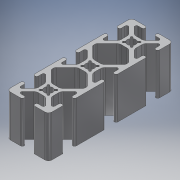
# Autodesk Inventor part: 1030-S
Saved by Autodesk Inventor 2017 SP1 (Build 210196100, 196)
## iProperties
Created: 2016-09-13
Part Number: 1030-S
Material: 6105-T5
Description: 40 S SHORT SINGLE UNIBEARING ASSEMBLY ON 40-4040 X 75mm
Document SubType Name: Modeling
Designer: BRALEF
Density: 1 g/cm^3
Appearance: CLEAR ANODIZED
MATERIAL: 6061-T6
PART PRICE: 44.65
Author: BRALEF
Autodesk Inventor part; units mm, degrees
ref_plane "YZ Plane" through (0, 0, 0) normal (1, 0, 0) x (0, 1, 0)
ref_plane "XZ Plane" through (0, 0, 0) normal (0, 1, 0) x (-1, 0, 0)
ref_plane "XY Plane" through (0, 0, 0) normal (0, 0, 1) x (1, 0, 0)
sketch "Sketch1" plane through (0, 0, 0) normal (0, 1, 0) x (-1, 0, 0)
  arc A0 (-1.9692, 2.8605) -> (-2.8605, 1.9692) centre (-2.4696, 2.4696) ccw
  line L0 (-2.2319, 1.3405) -> (-2.8605, 1.9692)
  arc A1 (-2.2319, 1.3405) -> (-2.2319, -1.3405) centre (0, 0) ccw
  line L1 (-2.8605, -1.9692) -> (-2.2319, -1.3405)
  arc A2 (-2.8605, -1.9692) -> (-1.9692, -2.8605) centre (-2.4696, -2.4696) ccw
  line L2 (-1.3405, -2.2319) -> (-1.9692, -2.8605)
  arc A3 (-1.3405, -2.2319) -> (1.3405, -2.2319) centre (0, 0) ccw
  line L3 (1.9692, -2.8605) -> (1.3405, -2.2319)
  arc A4 (1.9692, -2.8605) -> (2.8605, -1.9692) centre (2.4696, -2.4696) ccw
  line L4 (2.2319, -1.3405) -> (2.8605, -1.9692)
  arc A5 (2.2319, -1.3405) -> (2.2319, 1.3405) centre (0, 0) ccw
  line L5 (2.8605, 1.9692) -> (2.2319, 1.3405)
  arc A6 (2.8605, 1.9692) -> (1.9692, 2.8605) centre (2.4696, 2.4696) ccw
  line L6 (1.3405, 2.2319) -> (1.9692, 2.8605)
  arc A7 (1.3405, 2.2319) -> (-1.3405, 2.2319) centre (0, 0) ccw
  line L7 (-1.9692, 2.8605) -> (-1.3405, 2.2319)
  arc A8 (2.2319, -26.7405) -> (2.2319, -24.0595) centre (0, -25.4) ccw
  line L8 (2.8605, -23.4308) -> (2.2319, -24.0595)
  arc A9 (2.8605, -23.4308) -> (1.9692, -22.5395) centre (2.4696, -22.9304) ccw
  line L9 (1.3405, -23.1681) -> (1.9692, -22.5395)
  arc A10 (1.3405, -23.1681) -> (-1.3405, -23.1681) centre (0, -25.4) ccw
  line L10 (-1.9692, -22.5395) -> (-1.3405, -23.1681)
  arc A11 (-1.9692, -22.5395) -> (-2.8605, -23.4308) centre (-2.4696, -22.9304) ccw
  line L11 (-2.2319, -24.0595) -> (-2.8605, -23.4308)
  arc A12 (-2.2319, -24.0595) -> (-2.2319, -26.7405) centre (0, -25.4) ccw
  line L12 (-2.8605, -27.3692) -> (-2.2319, -26.7405)
  arc A13 (-2.8605, -27.3692) -> (-1.9692, -28.2605) centre (-2.4696, -27.8696) ccw
  line L13 (-1.3405, -27.6319) -> (-1.9692, -28.2605)
  arc A14 (-1.3405, -27.6319) -> (1.3405, -27.6319) centre (0, -25.4) ccw
  line L14 (1.9692, -28.2605) -> (1.3405, -27.6319)
  arc A15 (1.9692, -28.2605) -> (2.8605, -27.3692) centre (2.4696, -27.8696) ccw
  line L15 (2.2319, -26.7405) -> (2.8605, -27.3692)
  arc A16 (-9.5718, -11.1342) -> (-10.033, -12.2478) centre (-8.4582, -12.2478) ccw
  line L16 (-10.033, -13.1522) -> (-10.033, -12.2478)
  arc A17 (-10.033, -13.1522) -> (-9.5718, -14.2658) centre (-8.4582, -13.1522) ccw
  line L17 (-3.8846, -19.9529) -> (-9.5718, -14.2658)
  arc A18 (-3.8846, -19.9529) -> (-1.6396, -20.8828) centre (-1.6396, -17.7078) ccw
  line L18 (1.6396, -20.8828) -> (-1.6396, -20.8828)
  arc A19 (1.6396, -20.8828) -> (3.8846, -19.9529) centre (1.6396, -17.7078) ccw
  line L19 (9.5718, -14.2658) -> (3.8846, -19.9529)
  arc A20 (9.5718, -14.2658) -> (10.033, -13.1522) centre (8.4582, -13.1522) ccw
  line L20 (10.033, -12.2478) -> (10.033, -13.1522)
  arc A21 (10.033, -12.2478) -> (9.5718, -11.1342) centre (8.4582, -12.2478) ccw
  line L21 (3.8846, -5.4471) -> (9.5718, -11.1342)
  arc A22 (3.8846, -5.4471) -> (1.6396, -4.5172) centre (1.6396, -7.6922) ccw
  line L22 (-1.6396, -4.5172) -> (1.6396, -4.5172)
  arc A23 (-1.6396, -4.5172) -> (-3.8846, -5.4471) centre (-1.6396, -7.6922) ccw
  line L23 (-9.5718, -11.1342) -> (-3.8846, -5.4471)
  arc A24 (-9.5718, 14.2658) -> (-10.033, 13.1522) centre (-8.4582, 13.1522) ccw
  line L24 (-10.033, 12.2478) -> (-10.033, 13.1522)
  arc A25 (-10.033, 12.2478) -> (-9.5718, 11.1342) centre (-8.4582, 12.2478) ccw
  line L25 (-3.8846, 5.4471) -> (-9.5718, 11.1342)
  arc A26 (-3.8846, 5.4471) -> (-1.6396, 4.5172) centre (-1.6396, 7.6922) ccw
  line L26 (1.6396, 4.5172) -> (-1.6396, 4.5172)
  arc A27 (1.6396, 4.5172) -> (3.8846, 5.4471) centre (1.6396, 7.6922) ccw
  line L27 (9.5718, 11.1342) -> (3.8846, 5.4471)
  arc A28 (9.5718, 11.1342) -> (10.033, 12.2478) centre (8.4582, 12.2478) ccw
  line L28 (10.033, 13.1522) -> (10.033, 12.2478)
  arc A29 (10.033, 13.1522) -> (9.5718, 14.2658) centre (8.4582, 13.1522) ccw
  line L29 (3.8846, 19.9529) -> (9.5718, 14.2658)
  arc A30 (3.8846, 19.9529) -> (1.6396, 20.8828) centre (1.6396, 17.7078) ccw
  line L30 (-1.6396, 20.8828) -> (1.6396, 20.8828)
  arc A31 (-1.6396, 20.8828) -> (-3.8846, 19.9529) centre (-1.6396, 17.7078) ccw
  line L31 (-9.5718, 14.2658) -> (-3.8846, 19.9529)
  arc A32 (-1.9692, 28.2605) -> (-2.8605, 27.3692) centre (-2.4696, 27.8696) ccw
  line L32 (-2.2319, 26.7405) -> (-2.8605, 27.3692)
  arc A33 (-2.2319, 26.7405) -> (-2.2319, 24.0595) centre (0, 25.4) ccw
  line L33 (-2.8605, 23.4308) -> (-2.2319, 24.0595)
  arc A34 (-2.8605, 23.4308) -> (-1.9692, 22.5395) centre (-2.4696, 22.9304) ccw
  line L34 (-1.3405, 23.1681) -> (-1.9692, 22.5395)
  arc A35 (-1.3405, 23.1681) -> (1.3405, 23.1681) centre (0, 25.4) ccw
  line L35 (1.9692, 22.5395) -> (1.3405, 23.1681)
  arc A36 (1.9692, 22.5395) -> (2.8605, 23.4308) centre (2.4696, 22.9304) ccw
  line L36 (2.2319, 24.0595) -> (2.8605, 23.4308)
  arc A37 (2.2319, 24.0595) -> (2.2319, 26.7405) centre (0, 25.4) ccw
  line L37 (2.8605, 27.3692) -> (2.2319, 26.7405)
  arc A38 (2.8605, 27.3692) -> (1.9692, 28.2605) centre (2.4696, 27.8696) ccw
  line L38 (1.3405, 27.6319) -> (1.9692, 28.2605)
  arc A39 (1.3405, 27.6319) -> (-1.3405, 27.6319) centre (0, 25.4) ccw
  line L39 (-1.9692, 28.2605) -> (-1.3405, 27.6319)
  arc A40 (4.3561, -35.8902) -> (4.3561, -38.1) centre (4.3561, -36.9951) ccw
  line L40 (4.3561, -35.8902) -> (6.4749, -35.8902)
  arc A41 (6.4749, -35.8902) -> (7.1933, -34.1558) centre (6.4749, -34.8742) ccw
  line L41 (7.1933, -34.1558) -> (3.8846, -30.8471)
  arc A42 (3.8846, -30.8471) -> (1.6396, -29.9172) centre (1.6396, -33.0922) ccw
  line L42 (1.6396, -29.9172) -> (-1.6396, -29.9172)
  arc A43 (-1.6396, -29.9172) -> (-3.8846, -30.8471) centre (-1.6396, -33.0922) ccw
  line L43 (-3.8846, -30.8471) -> (-7.1933, -34.1558)
  arc A44 (-7.1933, -34.1558) -> (-6.4749, -35.8902) centre (-6.4749, -34.8742) ccw
  line L44 (-6.4749, -35.8902) -> (-4.3561, -35.8902)
  arc A45 (-4.3561, -38.1) -> (-4.3561, -35.8902) centre (-4.3561, -36.9951) ccw
  line L45 (-4.3561, -38.1) -> (-10.5918, -38.1)
  arc A46 (-12.7, -35.9918) -> (-10.5918, -38.1) centre (-10.5918, -35.9918) ccw
  line L46 (-12.7, -35.9918) -> (-12.7, -29.7561)
  arc A47 (-10.4902, -29.7561) -> (-12.7, -29.7561) centre (-11.5951, -29.7561) ccw
  line L47 (-10.4902, -29.7561) -> (-10.4902, -31.8749)
  arc A48 (-10.4902, -31.8749) -> (-8.7558, -32.5933) centre (-9.4742, -31.8749) ccw
  line L48 (-8.7558, -32.5933) -> (-5.4471, -29.2846)
  arc A49 (-5.4471, -29.2846) -> (-4.5172, -27.0396) centre (-7.6922, -27.0396) ccw
  line L49 (-4.5172, -27.0396) -> (-4.5172, -23.7604)
  arc A50 (-4.5172, -23.7604) -> (-5.4471, -21.5154) centre (-7.6922, -23.7604) ccw
  line L50 (-5.4471, -21.5154) -> (-8.7558, -18.2067)
  arc A51 (-8.7558, -18.2067) -> (-10.4902, -18.9251) centre (-9.4742, -18.9251) ccw
  line L51 (-10.4902, -18.9251) -> (-10.4902, -21.0439)
  arc A52 (-12.7, -21.0439) -> (-10.4902, -21.0439) centre (-11.5951, -21.0439) ccw
  line L52 (-12.7, -21.0439) -> (-12.7, -4.3561)
  arc A53 (-10.4902, -4.3561) -> (-12.7, -4.3561) centre (-11.5951, -4.3561) ccw
  line L53 (-10.4902, -4.3561) -> (-10.4902, -6.4749)
  arc A54 (-10.4902, -6.4749) -> (-8.7558, -7.1933) centre (-9.4742, -6.4749) ccw
  line L54 (-8.7558, -7.1933) -> (-5.4471, -3.8846)
  arc A55 (-5.4471, -3.8846) -> (-4.5172, -1.6396) centre (-7.6922, -1.6396) ccw
  line L55 (-4.5172, -1.6396) -> (-4.5172, 1.6396)
  arc A56 (-4.5172, 1.6396) -> (-5.4471, 3.8846) centre (-7.6922, 1.6396) ccw
  line L56 (-5.4471, 3.8846) -> (-8.7558, 7.1933)
  arc A57 (-8.7558, 7.1933) -> (-10.4902, 6.4749) centre (-9.4742, 6.4749) ccw
  line L57 (-10.4902, 6.4749) -> (-10.4902, 4.3561)
  arc A58 (-12.7, 4.3561) -> (-10.4902, 4.3561) centre (-11.5951, 4.3561) ccw
  line L58 (-12.7, 4.3561) -> (-12.7, 21.0439)
  arc A59 (-10.4902, 21.0439) -> (-12.7, 21.0439) centre (-11.5951, 21.0439) ccw
  line L59 (-10.4902, 21.0439) -> (-10.4902, 18.9251)
  arc A60 (-10.4902, 18.9251) -> (-8.7558, 18.2067) centre (-9.4742, 18.9251) ccw
  line L60 (-8.7558, 18.2067) -> (-5.4471, 21.5154)
  arc A61 (-5.4471, 21.5154) -> (-4.5172, 23.7604) centre (-7.6922, 23.7604) ccw
  line L61 (-4.5172, 23.7604) -> (-4.5172, 27.0396)
  arc A62 (-4.5172, 27.0396) -> (-5.4471, 29.2846) centre (-7.6922, 27.0396) ccw
  line L62 (-5.4471, 29.2846) -> (-8.7558, 32.5933)
  arc A63 (-8.7558, 32.5933) -> (-10.4902, 31.8749) centre (-9.4742, 31.8749) ccw
  line L63 (-10.4902, 31.8749) -> (-10.4902, 29.7561)
  arc A64 (-12.7, 29.7561) -> (-10.4902, 29.7561) centre (-11.5951, 29.7561) ccw
  line L64 (-12.7, 29.7561) -> (-12.7, 35.9918)
  arc A65 (-10.5918, 38.1) -> (-12.7, 35.9918) centre (-10.5918, 35.9918) ccw
  line L65 (-10.5918, 38.1) -> (-4.3561, 38.1)
  arc A66 (-4.3561, 35.8902) -> (-4.3561, 38.1) centre (-4.3561, 36.9951) ccw
  line L66 (-4.3561, 35.8902) -> (-6.4749, 35.8902)
  arc A67 (-6.4749, 35.8902) -> (-7.1933, 34.1558) centre (-6.4749, 34.8742) ccw
  line L67 (-7.1933, 34.1558) -> (-3.8846, 30.8471)
  arc A68 (-3.8846, 30.8471) -> (-1.6396, 29.9172) centre (-1.6396, 33.0922) ccw
  line L68 (-1.6396, 29.9172) -> (1.6396, 29.9172)
  arc A69 (1.6396, 29.9172) -> (3.8846, 30.8471) centre (1.6396, 33.0922) ccw
  line L69 (3.8846, 30.8471) -> (7.1933, 34.1558)
  arc A70 (7.1933, 34.1558) -> (6.4749, 35.8902) centre (6.4749, 34.8742) ccw
  line L70 (6.4749, 35.8902) -> (4.3561, 35.8902)
  arc A71 (4.3561, 38.1) -> (4.3561, 35.8902) centre (4.3561, 36.9951) ccw
  line L71 (4.3561, 38.1) -> (10.5918, 38.1)
  arc A72 (12.7, 35.9918) -> (10.5918, 38.1) centre (10.5918, 35.9918) ccw
  line L72 (12.7, 35.9918) -> (12.7, 29.7561)
  arc A73 (10.4902, 29.7561) -> (12.7, 29.7561) centre (11.5951, 29.7561) ccw
  line L73 (10.4902, 29.7561) -> (10.4902, 31.8749)
  arc A74 (10.4902, 31.8749) -> (8.7558, 32.5933) centre (9.4742, 31.8749) ccw
  line L74 (8.7558, 32.5933) -> (5.4471, 29.2846)
  arc A75 (5.4471, 29.2846) -> (4.5172, 27.0396) centre (7.6922, 27.0396) ccw
  line L75 (4.5172, 27.0396) -> (4.5172, 23.7604)
  arc A76 (4.5172, 23.7604) -> (5.4471, 21.5154) centre (7.6922, 23.7604) ccw
  line L76 (5.4471, 21.5154) -> (8.7558, 18.2067)
  arc A77 (8.7558, 18.2067) -> (10.4902, 18.9251) centre (9.4742, 18.9251) ccw
  line L77 (10.4902, 18.9251) -> (10.4902, 21.0439)
  arc A78 (12.7, 21.0439) -> (10.4902, 21.0439) centre (11.5951, 21.0439) ccw
  line L78 (12.7, 21.0439) -> (12.7, 4.3561)
  arc A79 (10.4902, 4.3561) -> (12.7, 4.3561) centre (11.5951, 4.3561) ccw
  line L79 (10.4902, 4.3561) -> (10.4902, 6.4749)
  arc A80 (10.4902, 6.4749) -> (8.7558, 7.1933) centre (9.4742, 6.4749) ccw
  line L80 (8.7558, 7.1933) -> (5.4471, 3.8846)
  arc A81 (5.4471, 3.8846) -> (4.5172, 1.6396) centre (7.6922, 1.6396) ccw
  line L81 (4.5172, 1.6396) -> (4.5172, -1.6396)
  arc A82 (4.5172, -1.6396) -> (5.4471, -3.8846) centre (7.6922, -1.6396) ccw
  line L82 (5.4471, -3.8846) -> (8.7558, -7.1933)
  arc A83 (8.7558, -7.1933) -> (10.4902, -6.4749) centre (9.4742, -6.4749) ccw
  line L83 (10.4902, -6.4749) -> (10.4902, -4.3561)
  arc A84 (12.7, -4.3561) -> (10.4902, -4.3561) centre (11.5951, -4.3561) ccw
  line L84 (12.7, -4.3561) -> (12.7, -21.0439)
  arc A85 (10.4902, -21.0439) -> (12.7, -21.0439) centre (11.5951, -21.0439) ccw
  line L85 (10.4902, -21.0439) -> (10.4902, -18.9251)
  arc A86 (10.4902, -18.9251) -> (8.7558, -18.2067) centre (9.4742, -18.9251) ccw
  line L86 (8.7558, -18.2067) -> (5.4471, -21.5154)
  arc A87 (5.4471, -21.5154) -> (4.5172, -23.7604) centre (7.6922, -23.7604) ccw
  line L87 (4.5172, -23.7604) -> (4.5172, -27.0396)
  arc A88 (4.5172, -27.0396) -> (5.4471, -29.2846) centre (7.6922, -27.0396) ccw
  line L88 (5.4471, -29.2846) -> (8.7558, -32.5933)
  arc A89 (8.7558, -32.5933) -> (10.4902, -31.8749) centre (9.4742, -31.8749) ccw
  line L89 (10.4902, -31.8749) -> (10.4902, -29.7561)
  arc A90 (12.7, -29.7561) -> (10.4902, -29.7561) centre (11.5951, -29.7561) ccw
  line L90 (12.7, -29.7561) -> (12.7, -35.9918)
  arc A91 (10.5918, -38.1) -> (12.7, -35.9918) centre (10.5918, -35.9918) ccw
  line L91 (10.5918, -38.1) -> (4.3561, -38.1)
  point P0 (0, 0)
  dimension "d0" = 1.1049
  dimension "d1" = 2.1082
  dimension "d2" = 1.016
  dimension "d3" = 1.5748
  dimension "d4" = 3.175
  dimension "d5" = 0.635
  dimension "d6" = 2.6035
  dimension "d7" = 2.6035
  dimension "d8" = 2.6035
  dimension "d9" = 2.6035
  dimension "d10" = 2.6035
  dimension "d11" = 2.6035
  dimension "d12" = 2.6035
  dimension "d13" = 2.6035
  dimension "d14" = 2.6035
  dimension "d15" = 2.6035
  dimension "d16" = 0
  dimension "d17" = 90
  dimension "d18" = 90
  dimension "d19" = 45
  dimension "d20" = 45
  dimension "d21" = 45
  dimension "d22" = 135
  dimension "d23" = 45
  dimension "d24" = 135
  dimension "d25" = 45
  dimension "d26" = 90
  dimension "d27" = 90
  dimension "d28" = 45
  dimension "d29" = 135
  dimension "d30" = 135
  dimension "d31" = 45
  dimension "d32" = 45
  dimension "d33" = 135
  dimension "d34" = 45
  dimension "d35" = 45
  dimension "d36" = 45
  dimension "d37" = 45
  dimension "d38" = 45
  dimension "d39" = 135
  dimension "d40" = 135
  dimension "d41" = 45
  dimension "d42" = 45
  dimension "d43" = 135
  dimension "d44" = 45
  dimension "d45" = 45
  dimension "d46" = 0
  dimension "d47" = 0
  dimension "d48" = 0
  dimension "d49" = 0
  dimension "d50" = 0
  dimension "d51" = 0
  dimension "d52" = 0
  dimension "d53" = 0
  dimension "d54" = 0
  dimension "d55" = 0
  dimension "d56" = 0
  dimension "d57" = 0
  dimension "d58" = 0
  dimension "d59" = 0
  dimension "d60" = 0
  dimension "d61" = 0
  dimension "d62" = 0
  dimension "d63" = 0
  constraints: 184 end point, 184 point on circle, 136 tangent, 92 centre point, 64 equal radius, 38 parallel, 1 horizontal, 1 perpendicular, 1 vertical
  measures "d0" radius of A73
  measures "d1" radius of A72
  measures "d2" radius of A74
  measures "d3" radius of A29
  measures "d4" radius of A75
  measures "d5" radius of A38
  measures "d6" radius of A37
  measures "d7" radius of A35
  measures "d8" radius of A39
  measures "d9" radius of A33
  measures "d10" radius of A7
  measures "d11" radius of A5
  measures "d12" radius of A1
  measures "d13" radius of A12
  measures "d14" radius of A14
  measures "d15" radius of A8
  measures "d16" angle of L20 L72
  measures "d17" angle of L71 L72
  measures "d18" angle of L91 L72
  measures "d19" angle of L72 L74
  measures "d20" angle of L72 L76
  measures "d21" angle of L72 L21
  measures "d22" angle of L72 L19
  measures "d23" angle of L72 L29
  measures "d24" angle of L72 L27
  measures "d25" angle of L72 L41
  measures "d26" angle of L72 L70
  measures "d27" angle of L72 L40
  measures "d28" angle of L72 L37
  measures "d29" angle of L72 L5
  measures "d30" angle of L72 L8
  measures "d31" angle of L72 L15
  measures "d32" angle of L72 L38
  measures "d33" angle of L72 L6
  measures "d34" angle of L72 L14
  measures "d35" angle of L72 L39
  measures "d36" angle of L72 L7
  measures "d37" angle of L72 L32
  measures "d38" angle of L72 L0
  measures "d39" angle of L72 L12
  measures "d40" angle of L72 L43
  measures "d41" angle of L72 L31
  measures "d42" angle of L72 L25
  measures "d43" angle of L72 L23
  measures "d44" angle of L72 L17
  measures "d45" angle of L72 L60
  measures "d46" angle of L78 L20
  measures "d47" angle of L84 L20
  measures "d48" angle of L90 L20
  measures "d49" angle of L77 L20
  measures "d50" angle of L79 L20
  measures "d51" angle of L83 L20
  measures "d52" angle of L85 L20
  measures "d53" angle of L89 L20
  measures "d54" angle of L20 L81
  measures "d55" angle of L20 L87
  measures "d56" angle of L20 L55
  measures "d57" angle of L20 L49
  measures "d58" angle of L20 L16
  measures "d59" angle of L20 L59
  measures "d60" angle of L20 L57
  measures "d61" angle of L20 L53
  measures "d62" angle of L20 L51
  measures "d63" angle of L20 L47
extrude "Extrusion1" add sketch "Sketch1" along normal mid plane 25.4
body "Solid1"
